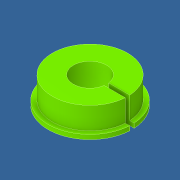
# Autodesk Inventor part: edingClamp
Saved by Autodesk Inventor 2016 (Build 200138000, 138)
## iProperties
Created: 2015-10-16
Part Number: edingClamp
Material: ABS-Kunststoff
Document SubType Name: Modeling
Designer: 4ndreas
Density: 1.06 g/cm^3
Appearance: Glatt - grün
Author: 4ndreas
Autodesk Inventor part; units mm, degrees
ref_plane "YZ Plane" through (0, 0, 0) normal (1, 0, 0) x (0, 1, 0)
ref_plane "XZ Plane" through (0, 0, 0) normal (0, 1, 0) x (-1, 0, 0)
ref_plane "XY Plane" through (0, 0, 0) normal (0, 0, 1) x (1, 0, 0)
sketch "Skizze1" plane through (0, 0, 0) normal (0, 0, 1) x (1, 0, 0)
  arc A0 (7.433, 1) -> (7.433, -1) centre (0, 0) ccw
  arc A1 (16.9706, 1) -> (16.9706, -1) centre (0, 0) ccw
  line L0 (0, 0) -> (15.5172, 0) construction
  line L1 (7.433, -1) -> (16.9706, -1)
  line L2 (7.433, 1) -> (16.9706, 1)
  circle A2 centre (0, 0) radius 7.5 construction
  circle A3 centre (0, 0) radius 17 construction
  dimension "d0" = 15
  dimension "d1" = 34
  dimension "d2" = 2
  constraints: 6 end point, 5 point on circle, 4 centre point, 4 coincident, 2 concentric, 1 horizontal, 1 parallel, 1 other
  measures "d0" diameter of A2
  measures "d1" diameter of A3
  measures "d2" distance between parallel lines of L1 L2
extrude "Extrusion1" add sketch "Skizze1" along normal blind 10
sketch "Skizze2" plane through (0, 0, 0) normal (0, 0, -1) x (-1, 0, 0)
  arc A0 (-7.433, -1) -> (-7.433, 1) centre (0, 0) ccw projected
  line L0 (-7.433, -1) -> (-16.9706, -1) projected
  arc A1 (-16.9706, -1) -> (-16.9706, 1) centre (0, 0) ccw projected
  line L1 (-16.9706, 1) -> (-7.433, 1) projected
  arc A2 (-18.9737, -1) -> (-18.9737, 1) centre (0, 0) ccw
  line L2 (-16.9706, -1) -> (-18.9737, -1)
  line L3 (-16.9706, 1) -> (-18.9737, 1)
  dimension "d5" = 2
  constraints: 4 end point, 2 point on circle, 1 centre point, 1 coincident, 1 collinear, 1 horizontal
  measures "d5" radial gap between concentric circles of A1 A2
extrude "Extrusion2" add sketch "Skizze2" along normal blind 2
